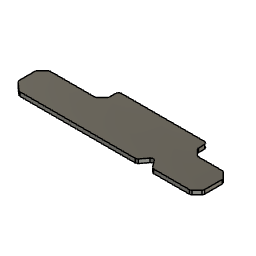
CNC-dreiebenk v11 (Autodesk Fusion 360 design; units mm, degrees)
Autodesk Fusion 360 part; units mm, degrees
note: some values were not read from the file. Set by a fixed rule: which sketch regions a step uses.
sketch "Sketch1" plane through (0, 0, 0) normal (0, 0, 1) x (1, 0, 0)
  line L0 (0, 0) -> (285, 0)
  line L1 (285, 0) -> (285, 50)
  line L2 (285, 50) -> (0, 50)
  line L3 (0, 50) -> (0, 0)
  line L4 (90.5213, 50) -> (225.5213, 50)
  line L5 (225.5213, 50) -> (225.5213, 75)
  line L6 (225.5213, 75) -> (90.5213, 75)
  line L7 (90.5213, 75) -> (90.5213, 50)
  line L8 (216.9969, 0) -> (193.0469, 0)
  line L9 (202.6853, -0.0546) -> (207.3953, -0.0546)
  line L10 (193.0469, 0) -> (205.0617, 15.8707)
  line L11 (205.0438, 15.8707) -> (216.9969, 0)
  circle A0 centre (140.3583, 38.3038) radius 18.9
  circle A1 centre (102.5213, 63.5005) radius 3.5
  circle A2 centre (118.2718, 63.2499) radius 2.25
  line L12 (111.8584, 9.8039) -> (168.8584, 9.8039)
  line L13 (168.8584, 9.8039) -> (168.8584, 66.8039)
  line L14 (168.8584, 66.8039) -> (111.8584, 66.8039)
  line L15 (111.8584, 66.8039) -> (111.8584, 9.8039)
  line L16 (14.2106, -0.0951) -> (-24.7294, -0.0951)
  line L17 (-24.7294, -0.0951) -> (-10.5221, 12.6845)
  line L18 (-10.5221, 12.6845) -> (-0.0196, 12.6845)
  line L19 (-0.0196, 12.6845) -> (14.2106, -0.0951)
  dimension "d1" = 285
  dimension "d2" = 50
  dimension "d7" = 135
  dimension "d8" = 25
  dimension "d36" = 23.95
  dimension "d37" = 4.71
  dimension "d41" = 37.8
  dimension "d42" = 7
  dimension "d43" = 4.5
  dimension "d45" = 57
  dimension "d46" = 57
  dimension "d52" = 38.94
  constraint horizontal L0
  constraint vertical L1
  constraint horizontal L2
  constraint vertical L3
  constraint coincident L0.start L3.end
  constraint horizontal L4
  constraint vertical L5
  constraint horizontal L6
  constraint vertical L7
  constraint coincident L2 L4.start
  constraint coincident L0 L8.start
  constraint horizontal L9
  constraint horizontal L12
  constraint vertical L13
  constraint horizontal L14
  constraint vertical L15
  constraint perpendicular L3 L16
  measures "d1" distance of L0.start L0.end
  measures "d2" distance of L0.start L2.end
  measures "d7" distance of L4.start L4.end
  measures "d8" distance of L4.start L6.end
  measures "d36" distance of L8.start L8.end
  measures "d37" distance of L9.start L9.end
  measures "d41" diameter of A0
  measures "d42" diameter of A1
  measures "d43" diameter of A2
  measures "d45" distance of L12.start L12.end
  measures "d46" distance of L12.start L14.end
  measures "d52" distance of L16.start L16.end
extrude "Extrude2" add sketch "Sketch1" along normal blind 6 contours L0 L1 L2 L3 L4 L10 L11 L12 L13 L15 L19 | L2 L4 L5 L6 L7 L13 L14 L15 | L2 L4 A0 L12 L13 L15 | L2 L4 A0 L13 L14 L15 | L2 L4 A0 | L2 L4 A0 | A1 | A2
chamfer "Chamfer9" distance 10 angle 45 5 edges at (285, 0, 3) (285, 50, 3) (225.5213, 50, 3) (90.5213, 50, 3) (0, 50, 3)
fillet "Fillet19" radius 4 17 edges at (216.9969, 0, 3) (193.0469, 0, 3) (205.0527, 15.8588, 3) (0, 12.667, 3) (14.1047, 0, 3) (0, 40, 3) (10, 50, 3) (90.5213, 60, 3) (80.5213, 50, 3) (225.5213, 60, 3) (235.5213, 50, 3) (275, 50, 3) (285, 40, 3) (285, 10, 3) (275, 0, 3) (90.5213, 75, 3) (225.5213, 75, 3)
equation "DBigHull = 3.78 cm"
equation "AvstandFraLangKantTilBigHull = 12.32 cm"
equation "motorfront = 56 mm"
equation "d41 = DBigHull"
equation "NEM23 = 57 mm"
equation "d45 = NEM23"
equation "d46 = NEM23"
